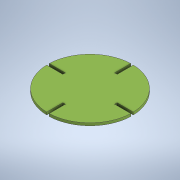
# Autodesk Inventor part: standin_hub
Saved by Autodesk Inventor 2021 (Build 250183000, 183)
## iProperties
Created: 2020-10-19
Part Number: standin_hub
Material: Generic
Document SubType Name: Modeling
Designer: dsouthall
Density: 1 g/cm^3
Appearance: Default
Author: dsouthall
Autodesk Inventor part; units mm, degrees
ref_plane "YZ Plane" through (0, 0, 0) normal (1, 0, 0) x (0, 1, 0)
ref_plane "XZ Plane" through (0, 0, 0) normal (0, 1, 0) x (-1, 0, 0)
ref_plane "XY Plane" through (0, 0, 0) normal (0, 0, 1) x (1, 0, 0)
sketch "Sketch1" plane through (0, 0, 0) normal (0, 1, 0) x (-1, 0, 0)
  point P0 (0, 0)
sketch "Sketch2" plane through (0, 0, 0) normal (0, 1, 0) x (-1, 0, 0)
  line L0 (46.5779, 0.8) -> (15.98, 0.8) construction
  line L1 (47.5028, -0.8) -> (-15.98, -0.8) construction
  line L2 (0.8, 38.8593) -> (0.8, 25.9877) construction
  line L3 (-0.8, 36.7319) -> (-0.8, -46.7895) construction
  arc A0 (15.98, 0.8) -> (0.8, 15.98) centre (0, 0) ccw construction
  arc A1 (-0.8, 15.98) -> (-15.98, 0.8) centre (0, 0) ccw construction
  line L4 (0.8, 25.9877) -> (0.8, -15.98) construction
  arc A2 (-0.8, 25.9877) -> (-25.9877, 0.8) centre (0, 0) ccw
  line L5 (0.8, -15.98) -> (0.8, -47.3445) construction
  arc A3 (0.8, -25.9877) -> (25.9877, -0.8) centre (0, 0) ccw
  arc A4 (25.9877, 0.8) -> (0.8, 25.9877) centre (0, 0) ccw
  line L6 (15.98, 0.8) -> (-25.9877, 0.8) construction
  line L7 (-15.98, -0.8) -> (-25.9877, -0.8) construction
  line L8 (-25.9877, 0.8) -> (-44.4844, 0.8) construction
  line L9 (-25.9877, -0.8) -> (-44.0655, -0.8) construction
  arc A5 (-25.9877, -0.8) -> (-0.8, -25.9877) centre (0, 0) ccw
  arc A6 (-15.98, -0.8) -> (-0.8, -15.98) centre (0, 0) ccw construction
  arc A7 (0.8, -15.98) -> (15.98, -0.8) centre (0, 0) ccw construction
  circle A8 centre (0, 0) radius 16 construction
  circle A9 centre (0, 0) radius 26 construction
  line L10 (25.9877, -0.8) -> (15.98, -0.8)
  line L11 (15.98, -0.8) -> (15.98, 0.8)
  line L12 (15.98, 0.8) -> (25.9877, 0.8)
  line L13 (0.8, -25.9877) -> (0.8, -15.98)
  line L14 (0.8, -15.98) -> (-0.8, -15.98)
  line L15 (-0.8, -15.98) -> (-0.8, -25.9877)
  line L16 (-25.9877, -0.8) -> (-15.98, -0.8)
  line L17 (-15.98, -0.8) -> (-15.98, 0.8)
  line L18 (-15.98, 0.8) -> (-25.9877, 0.8)
  line L19 (-0.8, 25.9877) -> (-0.8, 15.98)
  line L20 (-0.8, 15.98) -> (0.8, 15.98)
  line L21 (0.8, 15.98) -> (0.8, 25.9877)
  dimension "d2" = 0.8
  dimension "d3" = 0.8
  dimension "d4" = 0.8
  dimension "d5" = 0.8
  dimension "d6" = 32
  dimension "d7" = 0
  dimension "d8" = 0
  dimension "d9" = 52
  dimension "d10" = 0
  dimension "d11" = 0
  dimension "d12" = 0
  constraints: 44 end point, 19 point on circle, 12 point on line, 10 centre point, 8 collinear, 6 horizontal, 4 coincident, 4 vertical
  measures "d2" distance from line of point (0, 0) L1
  measures "d3" distance from line of point (0, 0) L0
  measures "d4" distance from line of L3 point (0, 0)
  measures "d5" distance from line of point (0, 0) L2
  measures "d6" diameter of A8
  measures "d7" radial gap between concentric circles of A8 A0
  measures "d8" radial gap between concentric circles of A8 A7
  measures "d9" diameter of A9
  measures "d10" radial gap between concentric circles of A9 A4
  measures "d11" radial gap between concentric circles of A9 A2
  measures "d12" radial gap between concentric circles of A5 A9
extrude "Extrusion1" add sketch "Sketch2" along normal blind 1.6
equation "\"d3\" = d2"
equation "\"d4\" = d2"
equation "\"d5\" = d2"
body "Solid1"
